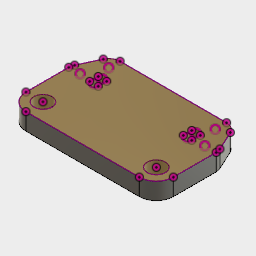
wire_strain_relief_vacuum (Autodesk Fusion 360 design; units mm, degrees)
Autodesk Fusion 360 part; units mm, degrees
sketch "Sketch1" plane through (0, 0, 0) normal (0, 1, 0) x (1, 0, 0)
  line L0 (-3, 0) -> (-3, 8)
  line L1 (-3, 8) -> (-0.6685, 13)
  line L2 (-0.6685, 13) -> (20.6685, 13)
  line L3 (20.6685, 13) -> (23, 8)
  line L4 (23, 8) -> (23, 0)
  line L5 (0, -3) -> (20, -3)
  arc A0 (-3, 0) -> (0, -3) centre (0, 0) ccw
  arc A1 (20, -3) -> (23, 0) centre (20, 0) ccw
  line L6 (10, -3) -> (10, 13) construction
  line L7 (1, 8.75) -> (1, 7.25)
  arc A2 (1, 7.25) -> (2.5, 7.25) centre (1.75, 7.25) ccw
  line L8 (2.5, 7.25) -> (2.5, 8.75)
  arc A3 (2.5, 8.75) -> (1, 8.75) centre (1.75, 8.75) ccw
  line L9 (1.75, 9.5) -> (1.75, 8) construction
  line L10 (17.5, 8.75) -> (17.5, 7.25)
  arc A4 (17.5, 7.25) -> (19, 7.25) centre (18.25, 7.25) ccw
  line L11 (19, 7.25) -> (19, 8.75)
  arc A5 (19, 8.75) -> (17.5, 8.75) centre (18.25, 8.75) ccw
  line L12 (18.25, 9.5) -> (18.25, 8) construction
  circle A6 centre (20, 0) radius 1.6
  circle A7 centre (0, 0) radius 1.6
  dimension "d1" = 20
  dimension "d2" = 6
  dimension "d3" = 8
  dimension "d4" = 5
  dimension "d5" = 65
  dimension "d6" = 15
  dimension "d7" = 8
  dimension "d8" = 3.2
  dimension "d10" = 1.5
  dimension "d11" = 1.5
  constraint coincident A0.centre A7.centre
  constraint equal A0 A1
  constraint vertical L0
  constraint horizontal L2
  constraint tangent L4 A1
  constraint vertical L4
  constraint tangent L5 A0
  constraint tangent L5 A1
  constraint midpoint L5 A0.centre
  constraint midpoint L2
  constraint horizontal L5
  constraint tangent L0 A0
  constraint tangent L7 A2
  constraint tangent A2 L8
  constraint parallel L7 L8
  constraint tangent L8 A3
  constraint tangent L7 A3
  constraint midpoint A3
  constraint midpoint A2 A0.centre
  constraint vertical L9
  constraint tangent L10 A4
  constraint tangent A4 L11
  constraint parallel L10 L11
  constraint tangent L11 A5
  constraint tangent L10 A5
  constraint midpoint A5
  constraint midpoint A4 A0.centre
  constraint parallel L6 L12
  constraint equal A2 A4
  constraint equal L8 L10
  constraint concentric A1 A6
  constraint equal A6 A7
  constraint horizontal A0.centre A7.centre
  measures "d2" diameter of A1
  measures "d4" distance of L2 A0.centre
  measures "d5" angle of L1 L5
  measures "d6" distance of L8 L10
  measures "d8" diameter of A7
  measures "d10" distance of L10 L11
  measures "d11" distance of A0.centre
extrude "Extrude1" add sketch "Sketch1" along normal blind 3
fillet "Fillet1" radius 2 4 edges at (23, 1.5, -8) (20.6685, 1.5, -13) (-0.6685, 1.5, -13) (-3, 1.5, -8)
ref_plane "WorkPlane1" through (10, 3, -5) normal (0, 1, 0) x (1, 0, 0)
sketch "Sketch2" plane through (10, 3, -4.5) normal (0, 1, 0) x (1, 0, 0)
  arc A0 (-12.8126, 3.9018) -> (-13, 3.0566) centre (-11, 3.0566) ccw
  line L0 (-13, 3.0566) -> (-13, -4.5)
  arc A1 (-13, -4.5) -> (-10, -7.5) centre (-10, -4.5) ccw
  line L1 (-10, -7.5) -> (10, -7.5)
  arc A2 (10, -7.5) -> (13, -4.5) centre (10, -4.5) ccw
  line L2 (13, -4.5) -> (13, 3.0566)
  arc A3 (13, 3.0566) -> (12.8126, 3.9018) centre (11, 3.0566) ccw
  line L3 (12.8126, 3.9018) -> (11.2069, 7.3452)
  arc A4 (11.2069, 7.3452) -> (9.3943, 8.5) centre (9.3943, 6.5) ccw
  line L4 (9.3943, 8.5) -> (-9.3943, 8.5)
  arc A5 (-9.3943, 8.5) -> (-11.2069, 7.3452) centre (-9.3943, 6.5) ccw
  line L5 (-11.2069, 7.3452) -> (-12.8126, 3.9018)
  circle A6 centre (10, -4.5) radius 1.6
  arc A7 (-7.5, 4.25) -> (-9, 4.25) centre (-8.25, 4.25) ccw
  line L6 (-7.5, 4.25) -> (-7.5, 2.75)
  arc A8 (-9, 2.75) -> (-7.5, 2.75) centre (-8.25, 2.75) ccw
  line L7 (-9, 2.75) -> (-9, 4.25)
  circle A9 centre (-10, -4.5) radius 1.6
  arc A10 (9, 4.25) -> (7.5, 4.25) centre (8.25, 4.25) ccw
  line L8 (9, 4.25) -> (9, 2.75)
  arc A11 (7.5, 2.75) -> (9, 2.75) centre (8.25, 2.75) ccw
  line L9 (7.5, 2.75) -> (7.5, 4.25)
